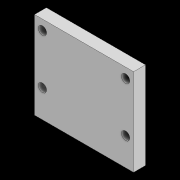
# Autodesk Inventor part: Sujetador_camara
Saved by Autodesk Inventor 2022 (Build 260153000, 153)
## iProperties
Created: 2021-10-20
Part Number: Sujetador_camara
Material: Genérico
Document SubType Name: Modeling
Designer: Julio R
Density: 1 g/cm^3
Appearance: Valor por defecto
Author: Julio R
Autodesk Inventor part; units mm, degrees
ref_plane "YZ Plane" through (0, 0, 0) normal (1, 0, 0) x (0, 1, 0)
ref_plane "XZ Plane" through (0, 0, 0) normal (0, 1, 0) x (-1, 0, 0)
ref_plane "XY Plane" through (0, 0, 0) normal (0, 0, 1) x (1, 0, 0)
sketch "Boceto1" plane through (0, 0, 0) normal (0, 0, 1) x (1, 0, 0)
  line L0 (0, 0) -> (25, 0)
  line L1 (25, 0) -> (25, 24)
  line L2 (25, 24) -> (0, 24)
  line L3 (0, 24) -> (0, 0)
  circle A0 centre (2, 2) radius 1.05
  circle A1 centre (23, 2) radius 1.05
  circle A2 centre (2, 14.5) radius 1.05
  circle A3 centre (23, 14.5) radius 1.05
  line L4 (0, 17) -> (25, 17)
  line L5 (0, 0) -> (25, 0)
  line L6 (25, 0) -> (25, -5)
  line L7 (25, -5) -> (0, -5)
  line L8 (0, -5) -> (0, 0)
  dimension "d0" = 25
  dimension "d1" = 24
  dimension "d2" = 2.1
  dimension "d3" = 2
  dimension "d4" = 2
  dimension "d7" = 21
  dimension "d10" = 12.5
  dimension "d13" = 7
  dimension "d14" = 5
  constraints: 18 end point, 4 centre point, 4 parallel, 3 horizontal, 3 perpendicular, 2 point on line, 1 vertical, 6 other
  measures "d0" distance of L2.end L1.end
  measures "d1" distance of L1.end L0.end
  measures "d2" diameter of A0
  measures "d3" horizontal distance of L0.start A0.centre
  measures "d4" distance from line of L3 A0.centre
  measures "d7" distance of A0.centre A1.centre
  measures "d10" distance of A0.centre A2.centre
  measures "d13" distance between parallel lines of L2 L4
  measures "d14" distance of L5.end L6.end
extrude "Extrusión1" add sketch "Boceto1" along normal blind 3 contours L3 L4 L1 L0 | L0 L6 L7 L8
